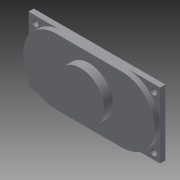
# Autodesk Inventor part: speaker
Saved by Autodesk Inventor 2016 (Build 200138000, 138)
## iProperties
Created: 2015-09-17
Part Number: speaker
Material: Generic
Document SubType Name: Modeling
Designer: Tyler
Density: 1 g/cm^3
Appearance: Default
Author: Tyler
Autodesk Inventor part; units mm, degrees
ref_plane "YZ Plane" through (0, 0, 0) normal (1, 0, 0) x (0, 1, 0)
ref_plane "XZ Plane" through (0, 0, 0) normal (0, 1, 0) x (-1, 0, 0)
ref_plane "XY Plane" through (0, 0, 0) normal (0, 0, 1) x (1, 0, 0)
sketch "Sketch1" plane through (0, 0, 0) normal (0, 1, 0) x (-1, 0, 0)
  line L0 (-20, 10) -> (20, 10)
  line L1 (20, 10) -> (20, -10)
  line L2 (20, -10) -> (-20, -10)
  line L3 (-20, -10) -> (-20, 10)
  point P0 (0, 0)
  dimension "d0" = 40
  dimension "d1" = 20
  dimension "d2" = 10
  dimension "d3" = 20
  constraints: 8 end point, 2 parallel, 1 horizontal, 1 perpendicular
  measures "d0" distance of L1.end L2.end
  measures "d1" distance of L0.end L1.end
  measures "d2" distance from line of point (0, 0) L0
  measures "d3" distance from line of L1 point (0, 0)
extrude "Extrusion1" add sketch "Sketch1" along normal blind 1.6
sketch "Sketch2" plane through (0, 0, 0) normal (0, -1, 0) x (1, 0, 0)
  line L0 (20, 10) -> (-20, 10) projected
  line L1 (-20, 10) -> (-20, -10) projected
  line L2 (-20, -10) -> (20, -10) projected
  line L3 (20, -10) -> (20, 10) projected
  line L4 (-10, 0) -> (10, 0) construction
  line L5 (-10, -10) -> (10, -10)
  line L6 (10, 10) -> (-10, 10)
  arc A0 (-10, 10) -> (-10, -10) centre (-10, 0) ccw
  arc A1 (10, -10) -> (10, 10) centre (10, 0) ccw
  point P0 (0, 0)
  point P1 (0, 0)
  dimension "d6" = 10
  constraints: 8 end point, 7 tangent, 4 point on circle, 2 centre point, 2 parallel, 1 midpoint
  measures "d6" radius of A1
extrude "Extrusion2" add sketch "Sketch2" along normal blind 1.6 contours A1 L2 A0 L0
sketch "Sketch3" plane through (0, -1.6, 0) normal (0, -1, 0) x (1, 0, 0)
  circle A0 centre (0, 0) radius 7.25
  dimension "d9" = 14.5
  constraints: 1 centre point, 1 coincident
  measures "d9" diameter of A0
extrude "Extrusion3" add sketch "Sketch3" along normal blind 2.6
sketch "Sketch4" plane through (0, 1.6, 0) normal (0, 1, 0) x (1, 0, 0)
  line L0 (-18, -8) -> (18, -8) construction
  line L1 (18, -8) -> (18, 8) construction
  line L2 (18, 8) -> (-18, 8) construction
  line L3 (-18, 8) -> (-18, -8) construction
  line L4 (-18, -8) -> (18, 8) construction
  line L5 (18, -8) -> (-18, 8) construction
  point P0 (0, 0)
  dimension "d12" = 36
  dimension "d13" = 16
  constraints: 12 end point, 4 coincident, 2 midpoint, 2 parallel, 1 horizontal, 1 perpendicular
  measures "d12" distance of L2.end L1.end
  measures "d13" distance of L1.end L0.end
hole "Hole1" at (-18, 1.6, -8) at (-18, 1.6, 8) at (18, 1.6, 8) at (18, 1.6, -8) direction (0, -1, 0) diameter 2 end through all
equation "\"d2\" = 0.5 * d1"
equation "\"d3\" = 0.5 * d0"
body "Solid1"
